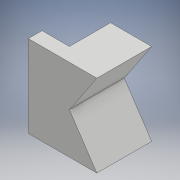
# Autodesk Inventor part: Part3
Saved by Autodesk Inventor 2018 (Build 220112000, 112)
## iProperties
Created: 2017-11-01
Part Number: Part3
Material: Generic
Document SubType Name: Modeling
Designer: kurtis
Density: 1 g/cm^3
Appearance: Default
Author: kurtis
Autodesk Inventor part; units mm, degrees
ref_plane "YZ Plane" through (0, 0, 0) normal (1, 0, 0) x (0, 1, 0)
ref_plane "XZ Plane" through (0, 0, 0) normal (0, 1, 0) x (-1, 0, 0)
ref_plane "XY Plane" through (0, 0, 0) normal (0, 0, 1) x (1, 0, 0)
sketch "Sketch3" plane through (0, 0, 0) normal (0, 0, 1) x (1, 0, 0)
  line L0 (0, 0) -> (-10, 0)
  line L1 (-25, 0) -> (-25, 5)
  line L2 (-25, 5) -> (-15, 5)
  line L3 (-15, 5) -> (-15, 20)
  line L4 (-15, 20) -> (-10, 20)
  line L5 (0, 20) -> (0, 0)
  line L6 (0, 20) -> (-10, 20)
  line L7 (-10, 20) -> (-10, 0)
  line L8 (-10, 20) -> (0, 20)
  line L9 (-10, 0) -> (-25, 0)
  line L10 (-25, 5) -> (-25, 20)
  line L11 (-25, 20) -> (-15, 20)
  dimension "d12" = 25
  dimension "d13" = 5
  dimension "d14" = 10
  dimension "d15" = 15
  dimension "d16" = 15
  dimension "d19" = 10
  constraints: 24 end point, 9 perpendicular, 2 horizontal, 1 vertical
  measures "d12" distance of L0.start L1.start
  measures "d13" distance of L1.start L1.end
  measures "d14" distance of L1.end L2.end
  measures "d15" distance of L2.end L3.end
  measures "d16" distance of L3.end L5.start
  measures "d19" distance of L5.start L4.end
extrude "Extrusion1" add sketch "Sketch3" along normal blind 15 contours L9 L1 L2 L3 L4 L7
extrude "Extrusion2" add sketch "Sketch3" against normal blind 15 contours L9 L1 L2 L3 L4 L7 | L3 L2 L10 L11
sketch "Sketch5" plane through (-25, 20, -15) normal (0, 1, 0) x (1, 0, 0)
  line L0 (15, 0) -> (15, -30) projected
  line L1 (15, 0) -> (15, -30)
  line L2 (15, -30) -> (25, -30)
  line L3 (25, -30) -> (15, -15)
  line L4 (15, 0) -> (25, 0)
  line L5 (25, 0) -> (15, -15)
  point P0 (25, -15)
  dimension "d24" = 10
  dimension "d25" = 10
  constraints: 10 end point, 1 horizontal, 1 midpoint, 1 perpendicular, 1 vertical
  measures "d24" distance of L0.end L2.end
  measures "d25" distance of L0.start L4.end
extrude "Extrusion4" add sketch "Sketch5" against normal blind 20
sketch "Sketch6" plane through (-25, 5, 15) normal (0, 1, 0) x (1, 0, 0)
  line L0 (0, 15) -> (0, 0) projected
  line L1 (10, 15) -> (0, 15)
  line L2 (0, 15) -> (10, 0)
  line L3 (10, 15) -> (0, 15) projected
  line L4 (10, 0) -> (10, 15)
  point P0 (25, 15)
  constraints: 6 end point, 1 horizontal, 1 perpendicular
extrude "Extrusion5" add sketch "Sketch6" along normal blind 10
body "Solid1"
